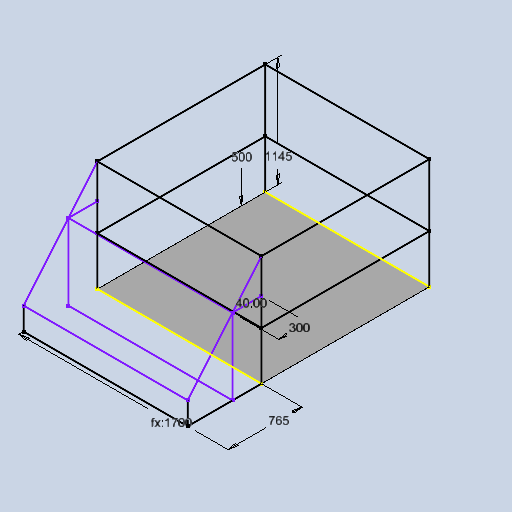
# Autodesk Inventor part: MSC DIM 009.1 BASE FRAME SKETCH
Saved by Autodesk Inventor 2025 (Build 290162010, 162A)
## iProperties
Created: 2024-05-19
Part Number: MSC DIM 009.1 BASE FRAME SKETCH
Material: Generic
Document SubType Name: Modeling
Designer: admin
Density: 1 g/cm^3
Appearance: Default
Stock Number: МОО DIM 009.1 эскиз базового основания
Author: admin
Autodesk Inventor part; units mm, degrees
ref_plane "YZ Plane" through (0, 0, 0) normal (1, 0, 0) x (0, 1, 0)
ref_plane "XZ Plane" through (0, 0, 0) normal (0, 1, 0) x (-1, 0, 0)
ref_plane "XY Plane" through (0, 0, 0) normal (0, 0, 1) x (1, 0, 0)
sketch "Sketch1" plane through (0, 0, 0) normal (0, 0, 1) x (1, 0, 0)
  line L0 (850, -1740) -> (-850, -1740)
  line L1 (-850, -1740) -> (-850, 0)
  line L2 (-850, 0) -> (850, 0)
  line L3 (850, 0) -> (850, -1740)
  line L4 (850, -1740) -> (-850, 0) construction
  line L5 (-850, -1740) -> (850, 0) construction
  point P0 (0, 0)
  point P1 (0, -870)
  point P2 (0, 0)
  dimension "d0" = 1700
  dimension "d1" = 1740
  constraints: 12 end point, 3 midpoint, 2 parallel, 1 coincident, 1 horizontal, 1 perpendicular
  measures "d0" distance of L1.end L2.end
  measures "d1" distance of L2.end L0.start
extrude "Extrusion1" add sketch "Sketch1" against normal blind 1
sketch3d "3D Sketch1"
equation "\"d8\" = d0"
body "Solid1"
